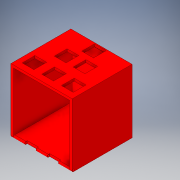
# Autodesk Inventor part: box final pt 1
Saved by Autodesk Inventor 2018 (Build 220112000, 112)
## iProperties
Created: 2019-09-18
Part Number: box final pt 1
Material: Generic
Document SubType Name: Modeling
Designer: 106282
Density: 1 g/cm^3
Appearance: Default
Author: 106282
Autodesk Inventor part; units mm, degrees
ref_plane "YZ Plane" through (0, 0, 0) normal (1, 0, 0) x (0, 1, 0)
ref_plane "XZ Plane" through (0, 0, 0) normal (0, 1, 0) x (-1, 0, 0)
ref_plane "XY Plane" through (0, 0, 0) normal (0, 0, 1) x (1, 0, 0)
sketch "Sketch1" plane through (0, 0, 0) normal (0, 0, 1) x (1, 0, 0)
  line L0 (0, 0) -> (152.4, 0)
  line L1 (152.4, 0) -> (152.4, 152.4)
  line L2 (152.4, 152.4) -> (0, 152.4)
  line L3 (0, 152.4) -> (0, 0)
  dimension "d0" = 152.4
  dimension "d1" = 152.4
  constraints: 8 end point, 2 parallel, 1 horizontal, 1 perpendicular
  measures "d0" distance of L2.end L1.end
  measures "d1" distance of L1.end L0.end
extrude "Extrusion1" add sketch "Sketch1" along normal blind 152.4
shell "Shell1" thickness 6.35 removed faces 1 at (101.6, 152.4, 50.8)
sketch "Sketch6" plane through (0, 0, 152.4) normal (0, 0, 1) x (1, 0, 0)
  line L0 (6.35, 152.4) -> (146.05, 152.4) projected
  line L1 (146.05, 6.35) -> (146.05, 152.4) projected
  line L2 (6.35, 152.4) -> (146.05, 152.4)
  line L3 (146.05, 152.4) -> (146.05, 6.35)
  line L4 (146.05, 6.35) -> (6.35, 6.35)
  line L5 (6.35, 6.35) -> (6.35, 152.4)
  point P0 (0, 0)
  constraints: 8 end point, 2 parallel, 1 horizontal, 1 perpendicular
extrude "Extrusion6" cut sketch "Sketch6" against normal blind 6.35
sketch "Sketch10" plane through (0, 0, 152.4) normal (0, 0, 1) x (1, 0, 0)
  line L0 (6.35, 152.4) -> (6.35, 6.35) projected
  line L1 (6.35, 6.35) -> (146.05, 6.35) projected
  line L2 (34.29, 6.35) -> (62.23, 6.35)
  line L3 (62.23, 6.35) -> (62.23, 0)
  line L4 (62.23, 0) -> (34.29, 0)
  line L5 (62.23, 0) -> (90.17, 0)
  line L6 (90.17, 0) -> (90.17, 6.35)
  line L7 (90.17, 6.35) -> (62.23, 6.35)
  line L8 (62.23, 6.35) -> (62.23, 0)
  line L9 (90.17, 6.35) -> (118.11, 6.35)
  line L10 (118.11, 6.35) -> (118.11, 0)
  line L11 (118.11, 0) -> (90.17, 0)
  line L12 (90.17, 0) -> (90.17, 6.35)
  line L13 (118.11, 0) -> (146.05, 0)
  line L14 (146.05, 0) -> (146.05, 6.35)
  line L15 (146.05, 6.35) -> (118.11, 6.35)
  line L16 (118.11, 6.35) -> (118.11, 0)
  line L17 (34.29, 0) -> (62.23, 0)
  line L18 (62.23, 0) -> (62.23, 6.35)
  line L19 (62.23, 6.35) -> (34.29, 6.35)
  line L20 (34.29, 6.35) -> (34.29, 0)
  line L21 (34.29, 6.35) -> (34.29, 0)
  line L22 (34.29, 0) -> (62.23, 0)
  line L23 (62.23, 0) -> (62.23, 6.35)
  line L24 (34.29, 6.35) -> (62.23, 6.35)
  dimension "d55" = 27.94
  dimension "d56" = 27.94
  dimension "d57" = 27.94
  dimension "d58" = 27.94
  constraints: 46 end point, 9 parallel, 7 perpendicular, 5 horizontal, 4 point on line
  measures "d55" distance of L3.end L4.end
  measures "d56" distance of L7.end L6.end
  measures "d57" distance of L10.end L11.end
  measures "d58" distance of L15.end L14.end
extrude "Extrusion10" cut sketch "Sketch10" against normal blind 6.35 contours L1 L3 L4 L20 | L1 L10 L11 L6
sketch "Sketch11" plane through (34.29, 0, 152.4) normal (1, 0, 0) x (0, 0, -1)
  circle A0 centre (3.175, 3.175) radius 2.54
  line L0 (0, 0) -> (0, 6.35) projected
  line L1 (6.35, 0) -> (0, 0) projected
  point P0 (152.4, 0)
  dimension "d61" = 5.08
  dimension "d62" = 3.175
  dimension "d63" = 3.175
  constraints: 1 centre point
  measures "d61" diameter of A0
  measures "d62" distance from line of L0 A0.centre
  measures "d63" distance from line of L1 A0.centre
extrude "Extrusion11" cut sketch "Sketch11" against normal blind 46.0375 and the other way blind 127
fillet "Fillet1" radius 3.175 6 edges at (20.32, 6.35, 152.4) (17.145, 0, 152.4) (76.2, 6.35, 152.4) (76.2, 0, 152.4) (132.08, 6.35, 152.4) (135.255, 0, 152.4)
sketch "Sketch12" plane through (0, 0, 0) normal (0, 0, -1) x (-1, 0, 0)
  line L0 (-152.4, 0) -> (-152.4, 152.4) projected
  line L1 (-152.4, 0) -> (0, 0)
  line L2 (0, 0) -> (0, 139.7)
  line L3 (0, 139.7) -> (-152.4, 139.7)
  line L4 (-152.4, 139.7) -> (-152.4, 0)
  dimension "d69" = 152.4
  dimension "d70" = 139.7
  constraints: 8 end point, 2 parallel, 1 horizontal, 1 perpendicular
  measures "d69" distance of L3.end L2.end
  measures "d70" distance of L2.end L1.end
extrude "Extrusion12" add sketch "Sketch12" along normal blind 88.9
shell "Shell2" thickness 6.35 removed faces 1 at (101.6, 93.1333, -88.9)
sketch "Sketch13" plane through (146.05, 133.35, 0) normal (0, 0, -1) x (-1, 0, 0)
  circle A0 centre (22.1223, -39.6694) radius 12.7
  point P0 (146.05, -133.35)
  dimension "d176" = 25.4
  constraints: 1 centre point
  measures "d176" diameter of A0
extrude "Extrusion13" cut sketch "Sketch13" against normal blind 50.8
sketch "Sketch14" plane through (0, 0, -88.9) normal (0, 0, -1) x (-1, 0, 0)
  point P0 (0, 0)
sketch "Sketch22" plane through (0, 152.4, 0) normal (0, 1, 0) x (1, 0, 0)
  line L0 (6.35, -152.4) -> (0, -152.4) projected
  line L1 (152.4, 0) -> (152.4, 88.9) projected
  line L2 (0, -152.4) -> (152.4, -152.4)
  line L3 (152.4, -152.4) -> (152.4, 0)
  line L4 (152.4, 0) -> (0, 0)
  line L5 (0, 0) -> (0, -152.4)
  constraints: 8 end point, 2 parallel, 1 horizontal, 1 perpendicular
extrude "Extrusion18" add sketch "Sketch22" along normal blind 6.35
sketch "Sketch23" plane through (0, 158.75, 0) normal (0, 1, 0) x (1, 0, 0)
  line L0 (38.1, -82.55) -> (67.31, -82.55)
  line L1 (67.31, -82.55) -> (67.31, -50.8)
  line L2 (67.31, -50.8) -> (38.1, -50.8)
  line L3 (12.7, -137.16) -> (41.91, -137.16)
  line L4 (41.91, -137.16) -> (41.91, -105.41)
  line L5 (41.91, -105.41) -> (12.7, -105.41)
  line L6 (12.7, -105.41) -> (12.7, -137.16)
  line L7 (110.49, -137.16) -> (139.7, -137.16)
  line L8 (139.7, -137.16) -> (139.7, -105.41)
  line L9 (139.7, -105.41) -> (110.49, -105.41)
  line L10 (110.49, -105.41) -> (110.49, -137.16)
  line L11 (114.3, -82.55) -> (114.3, -50.8)
  line L12 (61.595, -37.6132) -> (90.805, -37.6132)
  line L13 (90.805, -37.6132) -> (90.805, -5.8632)
  line L14 (90.805, -5.8632) -> (61.595, -5.8632)
  line L15 (61.595, -5.8632) -> (61.595, -37.6132)
  line L16 (61.595, -137.16) -> (90.805, -137.16)
  line L17 (90.805, -137.16) -> (90.805, -105.41)
  line L18 (90.805, -105.41) -> (61.595, -105.41)
  line L19 (61.595, -105.41) -> (61.595, -137.16)
  line L20 (0, 0) -> (0, -152.4) projected
  line L21 (152.4, -152.4) -> (152.4, 0) projected
  line L22 (0, -152.4) -> (152.4, -152.4) projected
  line L23 (152.4, 0) -> (0, 0) projected
  line L24 (38.1, -82.55) -> (38.1, -50.8)
  line L25 (114.3, -50.8) -> (85.09, -50.8)
  line L26 (85.09, -50.8) -> (85.09, -82.55)
  line L27 (85.09, -82.55) -> (114.3, -82.55)
  dimension "d120" = 29.21
  dimension "d121" = 31.75
  dimension "d122" = 29.21
  dimension "d123" = 31.75
  dimension "d128" = 29.21
  dimension "d129" = 31.75
  dimension "d130" = 12.7
  dimension "d131" = 12.7
  dimension "d132" = 19.685
  dimension "d133" = 15.24
  dimension "d134" = 15.24
  dimension "d135" = 15.24
  dimension "d136" = 50.8
  dimension "d142" = 38.1
  dimension "d143" = 38.1
  dimension "d144" = 29.21
  dimension "d145" = 50.8
  dimension "d147" = 29.21
  dimension "d148" = 31.75
  dimension "d149" = 61.595
  dimension "d150" = 29.21
  dimension "d151" = 31.75
  dimension "d152" = 31.75
  constraints: 48 end point, 9 parallel, 7 perpendicular, 6 horizontal, 1 vertical
  measures "d120" distance of L5.end L4.end
  measures "d121" distance of L4.end L3.end
  measures "d122" distance of L9.end L8.end
  measures "d123" distance of L8.end L7.end
  measures "d128" distance of L18.end L17.end
  measures "d129" distance of L17.end L16.end
  measures "d130" distance between parallel lines of L20 L6
  measures "d131" distance between parallel lines of L21 L8
  measures "d132" distance between parallel lines of L19 L4
  measures "d133" distance between parallel lines of L22 L3
  measures "d134" distance between parallel lines of L22 L16
  measures "d135" distance between parallel lines of L22 L7
  measures "d136" distance between parallel lines of L23 L2
  measures "d142" distance between parallel lines of L20 L24
  measures "d143" distance between parallel lines of L21 L11
  measures "d144" distance of L11.end L25.end
  measures "d145" distance between parallel lines of L23 L25
  measures "d147" distance of L13.end L14.end
  measures "d148" distance of L12.end L13.end
  measures "d149" distance between parallel lines of L21 L13
  measures "d150" distance of L1.end L2.end
  measures "d151" distance of L0.end L1.end
  measures "d152" distance of L11.start L11.end
extrude "Extrusion19" cut sketch "Sketch23" against normal blind 6.35 contours L24 L2 L1 L0 | L6 L5 L4 L3 | L10 L9 L8 L7 | L27 L26 L25 L11 | L15 L14 L13 L12 | L19 L18 L17 L16
sketch "Sketch27" plane through (0, 0, -88.9) normal (0, 0, -1) x (-1, 0, 0)
  line L0 (-62.23, 0) -> (-90.17, 0) projected
  line L1 (0, 139.7) -> (-152.4, 139.7) projected
  line L2 (-76.2, 139.7) -> (-76.2, 137.16)
  line L3 (-76.2, 0) -> (-76.2, 2.54)
  circle A0 centre (-76.2, 2.54) radius 1.397
  circle A1 centre (-76.2, 137.16) radius 1.397
  point P0 (0, 0)
  dimension "d169" = 2.54
  dimension "d170" = 2.54
  dimension "d171" = 2.794
  dimension "d172" = 2.794
  constraints: 4 end point, 2 centre point, 2 coincident, 2 midpoint, 2 vertical
  measures "d169" distance of L2.start L2.end
  measures "d170" distance of L3.start L3.end
  measures "d171" diameter of A0
  measures "d172" diameter of A1
extrude "Extrusion22" cut sketch "Sketch27" against normal blind 7.62
sketch "Sketch28" plane through (0, 0, -88.9) normal (0, 0, -1) x (-1, 0, 0)
  line L0 (37.6626, -24.8325) -> (-237.5642, -24.8325)
  line L1 (-237.5642, -24.8325) -> (-237.5642, 175.8968)
  line L2 (-237.5642, 175.8968) -> (37.6626, 175.8968)
  line L3 (37.6626, 175.8968) -> (37.6626, -24.8325)
  point P0 (0, 0)
  constraints: 8 end point, 2 parallel, 1 horizontal, 1 perpendicular
extrude "Extrusion23" cut sketch "Sketch28" against normal blind 92.075
body "Solid1"
